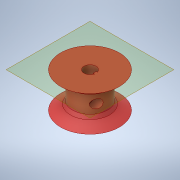
# Autodesk Inventor part: RoundShaftSpoolForArmV01
Saved by Autodesk Inventor 2022.2 (Build 262287010, 287A)
## iProperties
Created: 2019-02-24
Part Number: RoundShaftSpoolForArmV01
Material: PC/ABS Plastic
Document SubType Name: Modeling
Designer: steele
Density: 0.357273 g/cm^3
Appearance: Smooth - Red
holeForString: 0.200 in
stringDiameter: 0.120 in
clearanceForString: 0.080 in
clearanceForHexShaft: 0.020 in
spoolInteriorDiameter: 1.500 in
spoolInteriroRadius: 0.750 in
spoolExteriorDiameter: 2.500 in
spoolExteriorRadius: 1.250 in
hexHoleChamfer: 0.063 in
stringHoleCenterFromHexShaft: 0.360 in
textCircleDiameter: 1.875 in
textHeight: 0.180 in
textDepth: 0.050 in
Author: steele
Autodesk Inventor part; units mm, degrees
(part 1 of 2)
ref_plane "XZ Plane" through (0, 0, 0) normal (0, 1, 0) x (-1, 0, 0)
sketch "Sketch15" plane through (0, 0, 0) normal (0, 0, 1) x (1, 0, 0)
  line L0 (31.75, 0) -> (31.75, 76.2) construction
  line L1 (12.065, 0) -> (31.75, 0)
  line L2 (19.05, 0) -> (19.05, 76.2) construction
  line L3 (0, 76.2) -> (0, 0)
  line L4 (19.05, 19.05) -> (31.75, 19.05) construction
  line L5 (31.75, 0) -> (19.05, 7.3323)
  line L6 (31.75, 38.1) -> (19.05, 30.7677)
  line L7 (19.05, 30.7677) -> (31.75, 30.7677) construction
  line L8 (19.05, 30.7677) -> (19.05, 7.3323)
  line L9 (31.75, 38.1) -> (19.05, 45.4323)
  line L10 (19.05, 45.4323) -> (19.05, 68.8677)
  line L11 (19.05, 68.8677) -> (31.75, 76.2)
  line L12 (31.75, 38.1) -> (19.05, 38.1) construction
  line L13 (19.05, 68.8677) -> (31.75, 68.8677) construction
  line L14 (12.065, 0) -> (0, 0)
  line L15 (31.75, 76.2) -> (0, 76.2)
  dimension "d86" = 76.2
  dimension "d89" = 38.1
  dimension "centerLineForSpool" = 19.05
  dimension "d93" = 30
  dimension "d94" = 30
  dimension "d95" = 30
  dimension "d96" = 30
  dimension "d156" = 31.75
  dimension "d158" = 31.75
  constraints: 32 end point, 9 point on line, 3 horizontal, 2 midpoint, 2 perpendicular, 1 collinear, 1 vertical
  measures "d86" distance of L0.start L0.end
  measures "d89" distance from line of L6.start L1
  measures "centerLineForSpool" distance from line of L4.start L1
  measures "d93" angle of L5 L1
  measures "d94" angle of L6 L7
  measures "d95" angle of L9 L12
  measures "d96" angle of L11 L13
  measures "d156" distance from line of L0.end L3
  measures "d158" distance from line of L0.start L3
revolve "Revolution2" add sketch "Sketch15" angle 360 about axis through (0, 76.2, 0) along (0, -1, 0)
sketch "Sketch16" plane through (0, 0, 0) normal (0, -1, 0) x (1, 0, 0)
  line L0 (-7.6256, 0) -> (-3.8128, 6.604)
  line L1 (-3.8128, 6.604) -> (3.8128, 6.604)
  line L2 (3.8128, 6.604) -> (7.6256, 0)
  line L3 (7.6256, 0) -> (3.8128, -6.604)
  line L4 (3.8128, -6.604) -> (-3.8128, -6.604)
  line L5 (-3.8128, -6.604) -> (-7.6256, 0)
  point P0 (0, 0)
  point P1 (0, 0)
  dimension "d103" = 13.208
  constraints: 12 end point, 1 coincident, 1 horizontal, 13 other
  measures "d103" distance between parallel lines of L1 L4
extrude "Extrusion11" cut sketch "Sketch16" against normal through all
sketch "Sketch17" plane through (0, 0, 0) normal (1, 0, 0) x (0, 1, 0)
  circle A0 centre (57.15, 9.144) radius 2.54
  circle A1 centre (19.05, 9.144) radius 2.54
  line L0 (0, 31.75) -> (0, -31.75) projected
  line L1 (76.2, 31.75) -> (76.2, -31.75) projected
  line L2 (0, 6.604) -> (76.2, 6.604) projected
  point P0 (0, 0)
  point P1 (76.2, -31.75)
  point P2 (69.85, 6.858)
  point P3 (72.39, 6.858)
  dimension "d110" = 19.05
  dimension "d111" = 19.05
  dimension "d112" = 5.08
  constraints: 2 centre point, 1 equal radius, 4 other
  measures "d110" distance from line of A1.centre L0
  measures "d112" diameter of A0
extrude "Extrusion13" cut sketch "Sketch17" along normal through all both and the other way through all
ref_plane "Work Plane4" through (-19.05, 0, 0) normal (1, 0, 0) x (0, 1, 0)
sketch "Sketch22" plane through (-19.05, 0, 0) normal (1, 0, 0) x (0, 1, 0)
  spline S0 degree 8 poles (59.69, 9.144) (59.69, 9.42) (59.6557, 9.6896) (59.59, 9.9488) (59.4956, 10.1945) (59.3753, 10.4241) (59.2322, 10.6353) (59.069, 10.8263) (58.7143, 11.1594) (58.5223, 11.3044) (58.3151, 11.4282) (58.0956, 11.5293) (57.8665, 11.6061) (57.6306, 11.6579) (57.3908, 11.684) (56.8688, 11.684) (56.5895, 11.6484) (56.3166, 11.5781) (56.0542, 11.4743) (55.8066, 11.3384) (55.5778, 11.1726) (55.372, 10.9796) (55.0148, 10.5477) (54.8595, 10.305) (54.7334, 10.0377) (54.6415, 9.75) (54.5882, 9.4472) (54.5771, 9.1354) (54.6105, 8.8213) (54.8033, 8.0702) (55.0037, 7.6667) (55.2756, 7.316) (55.6042, 7.0287) (55.9734, 6.8124) (56.3659, 6.6712) (56.7636, 6.604) (57.4275, 6.604) (57.7064, 6.6386) (57.9825, 6.7085) (58.2515, 6.8141) (58.5088, 6.9552) (58.7493, 7.1318) (58.9675, 7.3429) (59.2831, 7.7498) (59.3961, 7.9265) (59.4931, 8.1154) (59.572, 8.3139) (59.6315, 8.5192) (59.6708, 8.7281) (59.69, 8.9374) (59.69, 9.144) knots 0 0 0 0 0 0 0 0 0 0.12897 0.12897 0.12897 0.12897 0.12897 0.12897 0.12897 0.253758 0.253758 0.253758 0.253758 0.253758 0.253758 0.253758 0.399502 0.399502 0.399502 0.399502 0.399502 0.399502 0.399502 0.544455 0.544455 0.544455 0.544455 0.544455 0.544455 0.544455 0.751871 0.751871 0.751871 0.751871 0.751871 0.751871 0.751871 0.90085 0.90085 0.90085 0.90085 0.90085 0.90085 0.90085 1 1 1 1 1 1 1 1 1 projected
  circle A0 centre (57.15, 9.144) radius 4.7625
  circle A1 centre (57.15, 9.144) radius 2.54 construction
  line L0 (57.15, 6.604) -> (19.05, 6.604) construction
  line L1 (76.2, 31.75) -> (76.2, -31.75) construction
  point P0 (0, 0)
  point P1 (69.85, 6.858)
  point P2 (76.2, -31.75)
  point P3 (72.39, 6.858)
  point P4 (19.05, 6.604)
  dimension "d121" = 19.05
  dimension "d122" = 5.08
  dimension "d125" = 9.525
  constraints: 2 centre point, 1 concentric, 1 vertical alignment, 3 other
  measures "d122" diameter of A1
  measures "d125" diameter of A0
extrude "Extrusion16" cut sketch "Sketch22" along normal blind 11.1125
ref_plane "Work Plane5" through (19.05, 0, 0) normal (1, 0, 0) x (0, 1, 0)
sketch "Sketch23" plane through (19.05, 0, 0) normal (1, 0, 0) x (0, 1, 0)
  line L0 (19.05, 6.604) -> (57.15, 6.604) projected
  circle A0 centre (19.05, 9.144) radius 2.54 construction
  line L1 (0, 31.75) -> (0, -31.75) projected
  circle A1 centre (19.05, 9.144) radius 4.7625
  point P0 (0, 0)
  dimension "d127" = 5.08
  dimension "d128" = 19.05
  dimension "d129" = 9.525
  constraints: 2 centre point, 1 coincident, 1 tangent
  measures "d127" diameter of A0
  measures "d128" distance from line of A0.centre L1
  measures "d129" diameter of A1
extrude "Extrusion17" cut sketch "Sketch23" against normal blind 11.1125
chamfer "Chamfer12" distance 2.3813 angle 45 4 edges at (-19.05, 68.8677, 0) (-19.05, 45.4323, 0) (-19.05, 30.7677, 0) (-19.05, 7.3323, 0)
ref_plane "Work Plane6" through (0, 38.1, 0) normal (0, -1, 0) x (1, 0, 0)
sketch "Sketch26" plane through (0, 0, 0) normal (0, -1, 0) x (1, 0, 0)
  circle A0 centre (0, 0) radius 23.8125 construction
  spline S0 degree 2 poles (-23.6535, 2.0269) (-23.7163, 1.1708) (-24.8247, 0.243) (-25.7608, 0.3118) knots 0 0 0 1 2 2 2
  spline S1 degree 2 poles (-25.7608, 0.3118) (-26.663, 0.378) (-27.6637, 1.4639) (-27.6008, 2.3199) knots 0 0 0 1 2 2 2
  spline S2 degree 2 poles (-27.6008, 2.3199) (-27.5843, 2.5447) (-27.5053, 2.9042) (-27.4499, 3.0673) knots 0 0 0 1 2 2 2
  spline S3 degree 2 poles (-27.4499, 3.0673) (-27.4004, 3.1937) (-27.2456, 3.4888) (-27.1893, 3.5806) knots 0 0 0 1 2 2 2
  line L0 (-27.1893, 3.5806) -> (-26.284, 3.5141)
  line L1 (-26.284, 3.5141) -> (-26.2911, 3.4187)
  spline S4 degree 2 poles (-26.2911, 3.4187) (-26.3578, 3.3524) (-26.5457, 3.1557) (-26.6354, 3.0291) knots 0 0 0 1 2 2 2
  spline S5 degree 2 poles (-26.6354, 3.0291) (-26.7283, 2.9028) (-26.8655, 2.594) (-26.8784, 2.4185) knots 0 0 0 1 2 2 2
  spline S6 degree 2 poles (-26.8784, 2.4185) (-26.8936, 2.2122) (-26.7894, 1.8609) (-26.6377, 1.6919) knots 0 0 0 1 2 2 2
  spline S7 degree 2 poles (-26.6377, 1.6919) (-26.5034, 1.5396) (-26.021, 1.3215) (-25.6853, 1.2969) knots 0 0 0 1 2 2 2
  spline S8 degree 2 poles (-25.6853, 1.2969) (-25.3312, 1.2709) (-24.834, 1.4232) (-24.6749, 1.5663) knots 0 0 0 1 2 2 2
  spline S9 degree 2 poles (-24.6749, 1.5663) (-24.5193, 1.7035) (-24.3664, 2.0576) (-24.353, 2.2392) knots 0 0 0 1 2 2 2
  spline S10 degree 2 poles (-24.353, 2.2392) (-24.3392, 2.4271) (-24.4404, 2.7781) (-24.5087, 2.9008) knots 0 0 0 1 2 2 2
  spline S11 degree 2 poles (-24.5087, 2.9008) (-24.5762, 3.0358) (-24.7252, 3.2418) (-24.7846, 3.3173) knots 0 0 0 1 2 2 2
  line L2 (-24.7846, 3.3173) -> (-24.7783, 3.4035)
  line L3 (-24.7783, 3.4035) -> (-23.8853, 3.338)
  spline S12 degree 2 poles (-23.8853, 3.338) (-23.8438, 3.2296) (-23.7407, 2.9465) (-23.7085, 2.7956) knots 0 0 0 1 2 2 2
  spline S13 degree 2 poles (-23.7085, 2.7956) (-23.6662, 2.6129) (-23.6336, 2.2978) (-23.6535, 2.0269) knots 0 0 0 1 2 2 2
  line L4 (-23.3485, 4.6994) -> (-23.5086, 3.8185)
  line L5 (-23.5086, 3.8185) -> (-26.3367, 4.3326)
  line L6 (-26.3367, 4.3326) -> (-26.1766, 5.2135)
  line L7 (-26.1766, 5.2135) -> (-23.3485, 4.6994)
  line L8 (-26.5756, 5.3143) -> (-26.7452, 4.3817)
  line L9 (-26.7452, 4.3817) -> (-27.4317, 4.5065)
  line L10 (-27.4317, 4.5065) -> (-27.2622, 5.4391)
  line L11 (-27.2622, 5.4391) -> (-26.5756, 5.3143)
  line L12 (-24.6721, 7.7572) -> (-24.6912, 7.6857)
  spline S14 degree 2 poles (-24.6912, 7.6857) (-24.7227, 7.6397) (-24.7907, 7.4565) (-24.8209, 7.3432) knots 0 0 0 1 2 2 2
  spline S15 degree 2 poles (-24.8209, 7.3432) (-24.8567, 7.2089) (-24.8566, 6.8861) (-24.8403, 6.7316) knots 0 0 0 1 2 2 2
  line L13 (-24.8403, 6.7316) -> (-22.9817, 6.2358)
  line L14 (-22.9817, 6.2358) -> (-23.2125, 5.3707)
  line L15 (-23.2125, 5.3707) -> (-25.9899, 6.1116)
  line L16 (-25.9899, 6.1116) -> (-25.7591, 6.9767)
  line L17 (-25.7591, 6.9767) -> (-25.3593, 6.8701)
  spline S16 degree 2 poles (-25.3593, 6.8701) (-25.3971, 6.9441) (-25.5085, 7.1975) (-25.5361, 7.2975) knots 0 0 0 1 2 2 2
  spline S17 degree 2 poles (-25.5361, 7.2975) (-25.5673, 7.4081) (-25.581, 7.6802) (-25.5516, 7.7905) knots 0 0 0 1 2 2 2
  spline S18 degree 2 poles (-25.5516, 7.7905) (-25.5405, 7.8323) (-25.5066, 7.9351) (-25.4925, 7.9761) knots 0 0 0 1 2 2 2
  line L18 (-25.4925, 7.9761) -> (-24.6721, 7.7572)
  spline S19 degree 2 poles (-22.0284, 8.846) (-22.1556, 8.5145) (-22.534, 8.028) (-22.7855, 7.8897) knots 0 0 0 1 2 2 2
  spline S20 degree 2 poles (-22.7855, 7.8897) (-23.0376, 7.7583) (-23.6514, 7.7358) (-24.0088, 7.8729) knots 0 0 0 1 2 2 2
  spline S21 degree 2 poles (-24.0088, 7.8729) (-24.3951, 8.0211) (-24.8413, 8.4701) (-24.9335, 8.7468) knots 0 0 0 1 2 2 2
  spline S22 degree 2 poles (-24.9335, 8.7468) (-25.0244, 9.0099) (-24.9779, 9.6138) (-24.8651, 9.9078) knots 0 0 0 1 2 2 2
  spline S23 degree 2 poles (-24.8651, 9.9078) (-24.78, 10.1298) (-24.5059, 10.5339) (-24.3072, 10.7156) knots 0 0 0 1 2 2 2
  line L19 (-24.3072, 10.7156) -> (-23.5923, 10.4413)
  line L20 (-23.5923, 10.4413) -> (-23.6332, 10.3347)
  spline S24 degree 2 poles (-23.6332, 10.3347) (-23.7021, 10.3016) (-23.8727, 10.2017) (-23.952, 10.1329) knots 0 0 0 1 2 2 2
  spline S25 degree 2 poles (-23.952, 10.1329) (-24.0393, 10.0606) (-24.1959, 9.8594) (-24.2501, 9.7181) knots 0 0 0 1 2 2 2
  spline S26 degree 2 poles (-24.2501, 9.7181) (-24.3728, 9.3982) (-24.0609, 8.8751) (-23.6804, 8.7291) knots 0 0 0 1 2 2 2
  spline S27 degree 2 poles (-23.6804, 8.7291) (-23.2768, 8.5743) (-22.7353, 8.7964) (-22.6158, 9.1077) knots 0 0 0 1 2 2 2
  spline S28 degree 2 poles (-22.6158, 9.1077) (-22.555, 9.2663) (-22.5364, 9.5303) (-22.5551, 9.6367) knots 0 0 0 1 2 2 2
  spline S29 degree 2 poles (-22.5551, 9.6367) (-22.572, 9.7391) (-22.6351, 9.9022) (-22.6618, 9.962) knots 0 0 0 1 2 2 2
  line L21 (-22.6618, 9.962) -> (-22.6209, 10.0687)
  line L22 (-22.6209, 10.0687) -> (-21.9031, 9.7933)
  spline S30 degree 2 poles (-21.9031, 9.7933) (-21.899, 9.7091) (-21.8902, 9.4907) (-21.9018, 9.3828) knots 0 0 0 1 2 2 2
  spline S31 degree 2 poles (-21.9018, 9.3828) (-21.9137, 9.2484) (-21.9609, 9.0218) (-22.0284, 8.846) knots 0 0 0 1 2 2 2
  line L23 (-20.3261, 12.4765) -> (-20.7511, 11.6885)
  line L24 (-20.7511, 11.6885) -> (-21.031, 11.8394)
  spline S32 degree 2 poles (-21.031, 11.8394) (-20.9697, 11.5433) (-20.975, 11.1041) (-21.1025, 10.8677) knots 0 0 0 1 2 2 2
  spline S33 degree 2 poles (-21.1025, 10.8677) (-21.3047, 10.4927) (-22.0074, 10.3279) (-22.4857, 10.5858) knots 0 0 0 1 2 2 2
  line L25 (-22.4857, 10.5858) -> (-24.1326, 11.4739)
  line L26 (-24.1326, 11.4739) -> (-23.7047, 12.2674)
  line L27 (-23.7047, 12.2674) -> (-22.4491, 11.5904)
  spline S34 degree 2 poles (-22.4491, 11.5904) (-22.2535, 11.4849) (-21.9932, 11.3691) (-21.8884, 11.3617) knots 0 0 0 1 2 2 2
  spline S35 degree 2 poles (-21.8884, 11.3617) (-21.7891, 11.3572) (-21.627, 11.4627) (-21.5537, 11.5986) knots 0 0 0 1 2 2 2
  spline S36 degree 2 poles (-21.5537, 11.5986) (-21.5098, 11.6801) (-21.4682, 11.9524) (-21.4875, 12.0856) knots 0 0 0 1 2 2 2
  line L28 (-21.4875, 12.0856) -> (-23.2811, 13.0528)
  line L29 (-23.2811, 13.0528) -> (-22.8561, 13.8409)
  line L30 (-22.8561, 13.8409) -> (-20.3261, 12.4765)
  line L31 (-19.4276, 13.7769) -> (-19.9318, 13.0369)
  line L32 (-19.9318, 13.0369) -> (-23.2209, 15.2776)
  line L33 (-23.2209, 15.2776) -> (-22.7167, 16.0176)
  line L34 (-22.7167, 16.0176) -> (-19.4276, 13.7769)
  spline S37 degree 2 poles (-18.2634, 15.7563) (-18.2637, 15.6357) (-18.2621, 15.4452) (-18.2941, 15.3109) knots 0 0 0 1 2 2 2
  spline S38 degree 2 poles (-18.2941, 15.3109) (-18.3264, 15.1809) (-18.4257, 14.966) (-18.5565, 14.8098) knots 0 0 0 1 2 2 2
  spline S39 degree 2 poles (-18.5565, 14.8098) (-18.8023, 14.5162) (-19.5183, 14.4593) (-19.8166, 14.7091) knots 0 0 0 1 2 2 2
  spline S40 degree 2 poles (-19.8166, 14.7091) (-20.0605, 14.9132) (-20.199, 15.3634) (-20.132, 15.6214) knots 0 0 0 1 2 2 2
  spline S41 degree 2 poles (-20.132, 15.6214) (-20.0654, 15.8837) (-19.7024, 16.4616) (-19.4716, 16.7758) knots 0 0 0 1 2 2 2
  line L35 (-19.4716, 16.7758) -> (-19.4834, 16.7857)
  spline S42 degree 2 poles (-19.4834, 16.7857) (-19.6657, 16.9383) (-20.0313, 16.7854) (-20.2573, 16.5155) knots 0 0 0 1 2 2 2
  spline S43 degree 2 poles (-20.2573, 16.5155) (-20.3584, 16.3947) (-20.5443, 15.9947) (-20.6044, 15.7833) knots 0 0 0 1 2 2 2
  line L36 (-20.6044, 15.7833) -> (-20.654, 15.7241)
  line L37 (-20.654, 15.7241) -> (-21.1867, 16.1701)
  spline S44 degree 2 poles (-21.1867, 16.1701) (-21.1298, 16.2957) (-20.8298, 16.8176) (-20.6356, 17.0496) knots 0 0 0 1 2 2 2
  spline S45 degree 2 poles (-20.6356, 17.0496) (-20.1599, 17.6178) (-19.3451, 17.8215) (-18.9568, 17.4965) knots 0 0 0 1 2 2 2
  line L38 (-18.9568, 17.4965) -> (-17.4583, 16.2419)
  line L39 (-17.4583, 16.2419) -> (-18.029, 15.5601)
  line L40 (-18.029, 15.5601) -> (-18.2634, 15.7563)
  line L41 (-18.6043, 16.0417) -> (-19.0613, 16.4242)
  spline S46 degree 2 poles (-19.0613, 16.4242) (-19.1913, 16.2352) (-19.3457, 15.9979) (-19.395, 15.862) knots 0 0 0 1 2 2 2
  spline S47 degree 2 poles (-19.395, 15.862) (-19.4415, 15.7439) (-19.3969, 15.5375) (-19.2927, 15.4503) knots 0 0 0 1 2 2 2
  spline S48 degree 2 poles (-19.2927, 15.4503) (-19.1388, 15.3215) (-18.8821, 15.3924) (-18.7454, 15.5558) knots 0 0 0 1 2 2 2
  spline S49 degree 2 poles (-18.7454, 15.5558) (-18.6701, 15.6458) (-18.5944, 15.9045) (-18.6043, 16.0417) knots 0 0 0 1 2 2 2
  line L42 (-16.9837, 19.5049) -> (-17.0374, 19.4538)
  spline S50 degree 2 poles (-17.0374, 19.4538) (-17.0882, 19.4311) (-17.2419, 19.3105) (-17.3269, 19.2296) knots 0 0 0 1 2 2 2
  spline S51 degree 2 poles (-17.3269, 19.2296) (-17.4276, 19.1339) (-17.5961, 18.8585) (-17.663, 18.7183) knots 0 0 0 1 2 2 2
  line L43 (-17.663, 18.7183) -> (-16.3373, 17.3245)
  line L44 (-16.3373, 17.3245) -> (-16.9861, 16.7074)
  line L45 (-16.9861, 16.7074) -> (-18.9671, 18.7902)
  line L46 (-18.9671, 18.7902) -> (-18.3183, 19.4073)
  line L47 (-18.3183, 19.4073) -> (-18.0332, 19.1075)
  spline S52 degree 2 poles (-18.0332, 19.1075) (-18.0268, 19.1904) (-17.9893, 19.4646) (-17.9606, 19.5643) knots 0 0 0 1 2 2 2
  spline S53 degree 2 poles (-17.9606, 19.5643) (-17.9295, 19.6749) (-17.799, 19.9141) (-17.7162, 19.9928) knots 0 0 0 1 2 2 2
  spline S54 degree 2 poles (-17.7162, 19.9928) (-17.6849, 20.0226) (-17.6023, 20.0926) (-17.5689, 20.1201) knots 0 0 0 1 2 2 2
  line L48 (-17.5689, 20.1201) -> (-16.9837, 19.5049)
  line L49 (-14.473, 22.9578) -> (-14.5289, 22.9193)
  spline S55 degree 2 poles (-14.5289, 22.9193) (-14.5809, 22.9022) (-14.7894, 22.8184) (-14.8682, 22.7641) knots 0 0 0 1 2 2 2
  spline S56 degree 2 poles (-14.8682, 22.7641) (-15.0919, 22.6099) (-15.1424, 22.335) (-14.9865, 22.1088) knots 0 0 0 1 2 2 2
  line L50 (-14.9865, 22.1088) -> (-14.9742, 22.091)
  line L51 (-14.9742, 22.091) -> (-14.387, 22.4959)
  line L52 (-14.387, 22.4959) -> (-14.033, 21.9824)
  line L53 (-14.033, 21.9824) -> (-14.5948, 21.5951)
  line L54 (-14.5948, 21.5951) -> (-13.3171, 19.742)
  line L55 (-13.3171, 19.742) -> (-14.0543, 19.2338)
  line L56 (-14.0543, 19.2338) -> (-15.3319, 21.0868)
  line L57 (-15.3319, 21.0868) -> (-15.6268, 20.8835)
  line L58 (-15.6268, 20.8835) -> (-15.9808, 21.397)
  line L59 (-15.9808, 21.397) -> (-15.6859, 21.6003)
  line L60 (-15.6859, 21.6003) -> (-15.7315, 21.6664)
  spline S57 degree 2 poles (-15.7315, 21.6664) (-16.0294, 22.0985) (-15.8724, 22.8443) (-15.4097, 23.1633) knots 0 0 0 1 2 2 2
  spline S58 degree 2 poles (-15.4097, 23.1633) (-15.2496, 23.2737) (-14.9568, 23.4419) (-14.8411, 23.4916) knots 0 0 0 1 2 2 2
  line L61 (-14.8411, 23.4916) -> (-14.473, 22.9578)
  spline S59 degree 2 poles (-10.6013, 22.9627) (-10.2664, 22.3365) (-10.5652, 21.2522) (-11.1887, 20.9187) knots 0 0 0 1 2 2 2
  spline S60 degree 2 poles (-11.1887, 20.9187) (-11.8094, 20.5867) (-12.8826, 20.9369) (-13.2176, 21.5631) knots 0 0 0 1 2 2 2
  spline S61 degree 2 poles (-13.2176, 21.5631) (-13.5555, 22.1947) (-13.2497, 23.2792) (-12.629, 23.6112) knots 0 0 0 1 2 2 2
  spline S62 degree 2 poles (-12.629, 23.6112) (-12.0083, 23.9433) (-10.9377, 23.5916) (-10.6013, 22.9627) knots 0 0 0 1 2 2 2
  spline S63 degree 2 poles (-11.407, 22.5247) (-11.5279, 22.7507) (-11.763, 23.0135) (-11.8764, 23.0684) knots 0 0 0 1 2 2 2
  spline S64 degree 2 poles (-11.8764, 23.0684) (-11.9982, 23.1258) (-12.2145, 23.1047) (-12.3261, 23.045) knots 0 0 0 1 2 2 2
  spline S65 degree 2 poles (-12.3261, 23.045) (-12.435, 22.9867) (-12.5715, 22.8296) (-12.5928, 22.6992) knots 0 0 0 1 2 2 2
  spline S66 degree 2 poles (-12.5928, 22.6992) (-12.6143, 22.5757) (-12.5314, 22.2243) (-12.4061, 21.9902) knots 0 0 0 1 2 2 2
  spline S67 degree 2 poles (-12.4061, 21.9902) (-12.2823, 21.7588) (-12.0532, 21.5137) (-11.944, 21.4601) knots 0 0 0 1 2 2 2
  spline S68 degree 2 poles (-11.944, 21.4601) (-11.8347, 21.4065) (-11.6005, 21.4267) (-11.4861, 21.4879) knots 0 0 0 1 2 2 2
  spline S69 degree 2 poles (-11.4861, 21.4879) (-11.3908, 21.5389) (-11.2385, 21.7254) (-11.2223, 21.8391) knots 0 0 0 1 2 2 2
  spline S70 degree 2 poles (-11.2223, 21.8391) (-11.2052, 21.9708) (-11.2788, 22.2851) (-11.407, 22.5247) knots 0 0 0 1 2 2 2
  line L62 (-8.4251, 24.4521) -> (-8.494, 24.4249)
  spline S71 degree 2 poles (-8.494, 24.4249) (-8.5496, 24.4229) (-8.7374, 24.3688) (-8.8465, 24.3257) knots 0 0 0 1 2 2 2
  spline S72 degree 2 poles (-8.8465, 24.3257) (-8.9758, 24.2747) (-9.2353, 24.0827) (-9.3498, 23.9778) knots 0 0 0 1 2 2 2
  line L63 (-9.3498, 23.9778) -> (-8.6439, 22.1885)
  line L64 (-8.6439, 22.1885) -> (-9.4769, 21.8599)
  line L65 (-9.4769, 21.8599) -> (-10.5317, 24.5338)
  line L66 (-10.5317, 24.5338) -> (-9.6988, 24.8624)
  line L67 (-9.6988, 24.8624) -> (-9.547, 24.4775)
  spline S73 degree 2 poles (-9.547, 24.4775) (-9.5099, 24.5519) (-9.3724, 24.792) (-9.3083, 24.8737) knots 0 0 0 1 2 2 2
  spline S74 degree 2 poles (-9.3083, 24.8737) (-9.2379, 24.9645) (-9.0273, 25.1373) (-8.921, 25.1792) knots 0 0 0 1 2 2 2
  spline S75 degree 2 poles (-8.921, 25.1792) (-8.8808, 25.1951) (-8.778, 25.229) (-8.7367, 25.242) knots 0 0 0 1 2 2 2
  line L68 (-8.7367, 25.242) -> (-8.4251, 24.4521)
  line L69 (-6.2391, 23.053) -> (-5.6856, 27.0364)
  line L70 (-5.6856, 27.0364) -> (-4.6604, 27.2312)
  line L71 (-4.6604, 27.2312) -> (-2.6841, 23.7286)
  line L72 (-2.6841, 23.7286) -> (-3.6517, 23.5447)
  line L73 (-3.6517, 23.5447) -> (-4.0306, 24.2647)
  line L74 (-4.0306, 24.2647) -> (-5.2075, 24.041)
  line L75 (-5.2075, 24.041) -> (-5.2988, 23.2317)
  line L76 (-5.2988, 23.2317) -> (-6.2391, 23.053)
  line L77 (-4.366, 24.9049) -> (-4.9834, 26.0699)
  line L78 (-4.9834, 26.0699) -> (-5.1334, 24.7591)
  line L79 (-5.1334, 24.7591) -> (-4.366, 24.9049)
  line L80 (-0.5268, 25.8575) -> (-0.6007, 25.8528)
  spline S76 degree 2 poles (-0.6007, 25.8528) (-0.6543, 25.8679) (-0.8496, 25.8739) (-0.9667, 25.8663) knots 0 0 0 1 2 2 2
  spline S77 degree 2 poles (-0.9667, 25.8663) (-1.1053, 25.8574) (-1.4112, 25.7542) (-1.5524, 25.6894) knots 0 0 0 1 2 2 2
  line L81 (-1.5524, 25.6894) -> (-1.4288, 23.7698)
  line L82 (-1.4288, 23.7698) -> (-2.3223, 23.7123)
  line L83 (-2.3223, 23.7123) -> (-2.5071, 26.5808)
  line L84 (-2.5071, 26.5808) -> (-1.6135, 26.6384)
  line L85 (-1.6135, 26.6384) -> (-1.5869, 26.2255)
  spline S78 degree 2 poles (-1.5869, 26.2255) (-1.5289, 26.2849) (-1.3243, 26.4713) (-1.2383, 26.5295) knots 0 0 0 1 2 2 2
  spline S79 degree 2 poles (-1.2383, 26.5295) (-1.1435, 26.5944) (-0.8901, 26.6942) (-0.7761, 26.7016) knots 0 0 0 1 2 2 2
  spline S80 degree 2 poles (-0.7761, 26.7016) (-0.7329, 26.7044) (-0.6247, 26.7051) (-0.5814, 26.7048) knots 0 0 0 1 2 2 2
  line L86 (-0.5814, 26.7048) -> (-0.5268, 25.8575)
  line L87 (3.3601, 23.6087) -> (3.4861, 25.0389)
  spline S81 degree 2 poles (3.4861, 25.0389) (3.5048, 25.2511) (3.5149, 25.5415) (3.4861, 25.6371) knots 0 0 0 1 2 2 2
  spline S82 degree 2 poles (3.4861, 25.6371) (3.4542, 25.7329) (3.3016, 25.83) (3.1571, 25.8427) knots 0 0 0 1 2 2 2
  spline S83 degree 2 poles (3.1571, 25.8427) (3.0556, 25.8517) (2.8509, 25.7798) (2.7267, 25.7071) knots 0 0 0 1 2 2 2
  line L88 (2.7267, 25.7071) -> (2.5481, 23.6802)
  line L89 (2.5481, 23.6802) -> (1.65, 23.7594)
  line L90 (1.65, 23.7594) -> (1.776, 25.1895)
  spline S84 degree 2 poles (1.776, 25.1895) (1.7945, 25.3987) (1.8017, 25.6925) (1.773, 25.788) knots 0 0 0 1 2 2 2
  spline S85 degree 2 poles (1.773, 25.788) (1.7411, 25.8838) (1.5885, 25.9809) (1.4439, 25.9937) knots 0 0 0 1 2 2 2
  spline S86 degree 2 poles (1.4439, 25.9937) (1.3363, 26.0031) (1.1151, 25.9203) (1.0105, 25.8583) knots 0 0 0 1 2 2 2
  line L91 (1.0105, 25.8583) -> (0.8319, 23.8314)
  line L92 (0.8319, 23.8314) -> (-0.06, 23.91)
  line L93 (-0.06, 23.91) -> (0.1923, 26.7734)
  line L94 (0.1923, 26.7734) -> (1.0842, 26.6948)
  line L95 (1.0842, 26.6948) -> (1.0563, 26.378)
  spline S87 degree 2 poles (1.0563, 26.378) (1.2909, 26.5433) (1.6999, 26.7181) (1.9429, 26.6967) knots 0 0 0 1 2 2 2
  spline S88 degree 2 poles (1.9429, 26.6967) (2.2043, 26.6736) (2.5822, 26.3893) (2.6648, 26.1309) knots 0 0 0 1 2 2 2
  spline S89 degree 2 poles (2.6648, 26.1309) (2.9412, 26.3484) (3.4192, 26.5666) (3.6529, 26.546) knots 0 0 0 1 2 2 2
  spline S90 degree 2 poles (3.6529, 26.546) (3.8529, 26.5284) (4.1585, 26.3744) (4.2548, 26.2357) knots 0 0 0 1 2 2 2
  spline S91 degree 2 poles (4.2548, 26.2357) (4.3626, 26.0868) (4.4492, 25.6979) (4.4223, 25.3934) knots 0 0 0 1 2 2 2
  line L96 (4.4223, 25.3934) -> (4.2581, 23.5296)
  line L97 (4.2581, 23.5296) -> (3.3601, 23.6087)
  line L98 (5.9237, 23.0684) -> (5.0434, 23.2767)
  line L99 (5.0434, 23.2767) -> (5.2751, 24.2561)
  line L100 (5.2751, 24.2561) -> (6.1555, 24.0479)
  line L101 (6.1555, 24.0479) -> (5.9237, 23.0684)
  line L102 (6.3538, 24.8862) -> (5.4734, 25.0944)
  line L103 (5.4734, 25.0944) -> (5.7052, 26.0739)
  line L104 (5.7052, 26.0739) -> (6.5855, 25.8657)
  line L105 (6.5855, 25.8657) -> (6.3538, 24.8862)
  spline S92 degree 2 poles (11.5194, 23.0401) (11.3241, 22.5864) (10.8864, 21.9681) (10.6258, 21.808) knots 0 0 0 1 2 2 2
  spline S93 degree 2 poles (10.6258, 21.808) (10.3693, 21.6495) (9.7559, 21.638) (9.3873, 21.7967) knots 0 0 0 1 2 2 2
  spline S94 degree 2 poles (9.3873, 21.7967) (9.0158, 21.9567) (8.6055, 22.409) (8.544, 22.7112) knots 0 0 0 1 2 2 2
  spline S95 degree 2 poles (8.544, 22.7112) (8.4812, 23.0105) (8.6272, 23.7477) (8.8226, 24.2014) knots 0 0 0 1 2 2 2
  spline S96 degree 2 poles (8.8226, 24.2014) (9.0228, 24.6665) (9.4508, 25.2621) (9.7178, 25.4295) knots 0 0 0 1 2 2 2
  spline S97 degree 2 poles (9.7178, 25.4295) (9.9824, 25.5912) (10.599, 25.5946) (10.9564, 25.4407) knots 0 0 0 1 2 2 2
  spline S98 degree 2 poles (10.9564, 25.4407) (11.3335, 25.2783) (11.7357, 24.8228) (11.796, 24.5178) knots 0 0 0 1 2 2 2
  spline S99 degree 2 poles (11.796, 24.5178) (11.8559, 24.2197) (11.7087, 23.4797) (11.5194, 23.0401) knots 0 0 0 1 2 2 2
  spline S100 degree 2 poles (10.6375, 23.4199) (10.9171, 24.0693) (10.9303, 24.6855) (10.678, 24.7942) knots 0 0 0 1 2 2 2
  spline S101 degree 2 poles (10.678, 24.7942) (10.4256, 24.9028) (9.9841, 24.471) (9.7033, 23.8188) knots 0 0 0 1 2 2 2
  spline S102 degree 2 poles (9.7033, 23.8188) (9.4273, 23.1779) (9.4133, 22.552) (9.6657, 22.4433) knots 0 0 0 1 2 2 2
  spline S103 degree 2 poles (9.6657, 22.4433) (9.9152, 22.3358) (10.3603, 22.7762) (10.6375, 23.4199) knots 0 0 0 1 2 2 2
  line L106 (12.0369, 20.5512) -> (11.2478, 20.9935)
  line L107 (11.2478, 20.9935) -> (11.74, 21.8715)
  line L108 (11.74, 21.8715) -> (12.5291, 21.4292)
  line L109 (12.5291, 21.4292) -> (12.0369, 20.5512)
  spline S104 degree 2 poles (15.6568, 19.6743) (15.4839, 19.4297) (15.0253, 19.1338) (14.7562, 19.1009) knots 0 0 0 1 2 2 2
  spline S105 degree 2 poles (14.7562, 19.1009) (14.4872, 19.068) (13.9226, 19.2213) (13.5948, 19.4529) knots 0 0 0 1 2 2 2
  spline S106 degree 2 poles (13.5948, 19.4529) (13.2486, 19.7013) (12.8296, 20.1676) (12.7174, 20.3566) knots 0 0 0 1 2 2 2
  line L110 (12.7174, 20.3566) -> (13.1967, 21.0348)
  line L111 (13.1967, 21.0348) -> (13.2673, 20.9849)
  spline S107 degree 2 poles (13.2673, 20.9849) (13.3046, 20.9094) (13.3903, 20.7203) (13.4767, 20.5912) knots 0 0 0 1 2 2 2
  spline S108 degree 2 poles (13.4767, 20.5912) (13.5574, 20.4699) (13.7458, 20.2498) (13.8845, 20.1518) knots 0 0 0 1 2 2 2
  spline S109 degree 2 poles (13.8845, 20.1518) (14.0055, 20.0662) (14.3307, 19.9272) (14.4735, 19.9473) knots 0 0 0 1 2 2 2
  spline S110 degree 2 poles (14.4735, 19.9473) (14.581, 19.9657) (14.7603, 20.0697) (14.8512, 20.1982) knots 0 0 0 1 2 2 2
  spline S111 degree 2 poles (14.8512, 20.1982) (14.9296, 20.3092) (14.9493, 20.5297) (14.9101, 20.6292) knots 0 0 0 1 2 2 2
  spline S112 degree 2 poles (14.9101, 20.6292) (14.8541, 20.7747) (14.58, 21.0289) (14.4716, 21.1055) knots 0 0 0 1 2 2 2
  spline S113 degree 2 poles (14.4716, 21.1055) (14.3001, 21.2267) (13.9357, 21.4011) (13.7958, 21.4546) knots 0 0 0 1 2 2 2
  line L112 (13.7958, 21.4546) -> (13.7277, 21.5027)
  line L113 (13.7277, 21.5027) -> (14.9626, 23.25)
  line L114 (14.9626, 23.25) -> (17.0251, 21.7924)
  line L115 (17.0251, 21.7924) -> (16.6099, 21.2049)
  line L116 (16.6099, 21.2049) -> (15.2862, 22.1404)
  line L117 (15.2862, 22.1404) -> (14.9209, 21.6235)
  spline S114 degree 2 poles (14.9209, 21.6235) (14.9875, 21.584) (15.165, 21.4661) (15.2129, 21.4322) knots 0 0 0 1 2 2 2
  spline S115 degree 2 poles (15.2129, 21.4322) (15.4373, 21.2736) (15.7514, 20.9156) (15.8342, 20.7172) knots 0 0 0 1 2 2 2
  spline S116 degree 2 poles (15.8342, 20.7172) (15.9287, 20.4764) (15.8528, 19.9517) (15.6568, 19.6743) knots 0 0 0 1 2 2 2
  line L118 (17.4262, 16.2992) -> (15.3871, 18.2186)
  line L119 (15.3871, 18.2186) -> (15.8124, 18.6705)
  spline S117 degree 2 poles (15.8124, 18.6705) (16.2657, 18.634) (17.0222, 18.6088) (17.3318, 18.6269) knots 0 0 0 1 2 2 2
  spline S118 degree 2 poles (17.3318, 18.6269) (17.7374, 18.6479) (18.2264, 18.8025) (18.3872, 18.9734) knots 0 0 0 1 2 2 2
  spline S119 degree 2 poles (18.3872, 18.9734) (18.5692, 19.1667) (18.5323, 19.5915) (18.3255, 19.7862) knots 0 0 0 1 2 2 2
  spline S120 degree 2 poles (18.3255, 19.7862) (18.2198, 19.8857) (17.9823, 20.0117) (17.8475, 20.0623) knots 0 0 0 1 2 2 2
  spline S121 degree 2 poles (17.8475, 20.0623) (17.7129, 20.1084) (17.4933, 20.1455) (17.4385, 20.1547) knots 0 0 0 1 2 2 2
  line L120 (17.4385, 20.1547) -> (17.3845, 20.2055)
  line L121 (17.3845, 20.2055) -> (17.9538, 20.8103)
  spline S122 degree 2 poles (17.9538, 20.8103) (18.1236, 20.7565) (18.7327, 20.4036) (18.9643, 20.1856) knots 0 0 0 1 2 2 2
  spline S123 degree 2 poles (18.9643, 20.1856) (19.4589, 19.72) (19.5522, 18.8011) (19.1776, 18.4032) knots 0 0 0 1 2 2 2
  spline S124 degree 2 poles (19.1776, 18.4032) (18.947, 18.1581) (18.271, 17.904) (17.7495, 17.886) knots 0 0 0 1 2 2 2
  spline S125 degree 2 poles (17.7495, 17.886) (17.4243, 17.8784) (16.864, 17.9182) (16.7435, 17.9298) knots 0 0 0 1 2 2 2
  line L122 (16.7435, 17.9298) -> (17.9193, 16.8231)
  line L123 (17.9193, 16.8231) -> (17.4262, 16.2992)
  spline S126 degree 2 poles (20.9848, 14.9394) (20.5993, 14.6304) (19.9226, 14.2898) (19.6174, 14.2707) knots 0 0 0 1 2 2 2
  spline S127 degree 2 poles (19.6174, 14.2707) (19.3166, 14.2511) (18.7695, 14.5288) (18.5184, 14.842) knots 0 0 0 1 2 2 2
  spline S128 degree 2 poles (18.5184, 14.842) (18.2655, 15.1576) (18.1154, 15.7496) (18.2029, 16.0453) knots 0 0 0 1 2 2 2
  spline S129 degree 2 poles (18.2029, 16.0453) (18.288, 16.339) (18.7628, 16.9215) (19.1483, 17.2304) knots 0 0 0 1 2 2 2
  spline S130 degree 2 poles (19.1483, 17.2304) (19.5434, 17.5471) (20.2008, 17.8723) (20.5152, 17.8948) knots 0 0 0 1 2 2 2
  spline S131 degree 2 poles (20.5152, 17.8948) (20.8247, 17.9134) (21.3708, 17.627) (21.6141, 17.3235) knots 0 0 0 1 2 2 2
  spline S132 degree 2 poles (21.6141, 17.3235) (21.871, 17.003) (22.0123, 16.412) (21.9224, 16.1144) knots 0 0 0 1 2 2 2
  spline S133 degree 2 poles (21.9224, 16.1144) (21.8355, 15.8231) (21.3582, 15.2387) (20.9848, 14.9394) knots 0 0 0 1 2 2 2
  spline S134 degree 2 poles (20.3842, 15.6886) (20.9359, 16.1308) (21.2367, 16.6688) (21.0649, 16.8832) knots 0 0 0 1 2 2 2
  spline S135 degree 2 poles (21.0649, 16.8832) (20.893, 17.0976) (20.3005, 16.9234) (19.7465, 16.4793) knots 0 0 0 1 2 2 2
  spline S136 degree 2 poles (19.7465, 16.4793) (19.202, 16.0428) (18.8959, 15.4967) (19.0677, 15.2823) knots 0 0 0 1 2 2 2
  spline S137 degree 2 poles (19.0677, 15.2823) (19.2377, 15.0703) (19.8373, 15.2503) (20.3842, 15.6886) knots 0 0 0 1 2 2 2
  line L124 (21.5114, 10.2638) -> (20.5498, 12.0744)
  line L125 (20.5498, 12.0744) -> (21.1361, 12.3858)
  line L126 (21.1361, 12.3858) -> (21.3924, 11.9031)
  line L127 (21.3924, 11.9031) -> (23.5848, 13.0674)
  line L128 (23.5848, 13.0674) -> (23.3284, 13.5501)
  line L129 (23.3284, 13.5501) -> (23.9147, 13.8615)
  line L130 (23.9147, 13.8615) -> (24.8763, 12.0508)
  line L131 (24.8763, 12.0508) -> (24.29, 11.7395)
  line L132 (24.29, 11.7395) -> (24.0337, 12.2221)
  line L133 (24.0337, 12.2221) -> (21.8413, 11.0578)
  line L134 (21.8413, 11.0578) -> (22.0977, 10.5751)
  line L135 (22.0977, 10.5751) -> (21.5114, 10.2638)
  spline S138 degree 2 poles (24.7622, 7.1655) (24.2608, 6.9813) (23.3117, 7.1294) (22.9778, 7.385) knots 0 0 0 1 2 2 2
  spline S139 degree 2 poles (22.9778, 7.385) (22.6959, 7.5973) (22.351, 8.2139) (22.2158, 8.582) knots 0 0 0 1 2 2 2
  line L136 (22.2158, 8.582) -> (21.8049, 9.7007)
  line L137 (21.8049, 9.7007) -> (25.3813, 11.0143)
  line L138 (25.3813, 11.0143) -> (25.788, 9.9071)
  spline S140 degree 2 poles (25.788, 9.9071) (25.9263, 9.5304) (26.0723, 8.8373) (25.9933, 8.4794) knots 0 0 0 1 2 2 2
  spline S141 degree 2 poles (25.9933, 8.4794) (25.896, 8.0457) (25.281, 7.356) (24.7622, 7.1655) knots 0 0 0 1 2 2 2
  spline S142 degree 2 poles (24.4295, 8.0892) (24.7831, 8.2191) (25.198, 8.6478) (25.2484, 8.9492) knots 0 0 0 1 2 2 2
  spline S143 degree 2 poles (25.2484, 8.9492) (25.2799, 9.168) (25.1533, 9.5754) (25.0511, 9.8536) knots 0 0 0 1 2 2 2
  line L139 (25.0511, 9.8536) -> (25.0447, 9.871)
  line L140 (25.0447, 9.871) -> (22.8044, 9.0482)
  line L141 (22.8044, 9.0482) -> (22.8108, 9.0308)
  spline S144 degree 2 poles (22.8108, 9.0308) (22.9215, 8.7294) (23.094, 8.3224) (23.282, 8.1776) knots 0 0 0 1 2 2 2
  spline S145 degree 2 poles (23.282, 8.1776) (23.502, 8.0084) (24.0759, 7.9594) (24.4295, 8.0892) knots 0 0 0 1 2 2 2
  line L142 (25.1133, 5.3864) -> (24.908, 6.2674)
  line L143 (24.908, 6.2674) -> (25.8883, 6.4959)
  line L144 (25.8883, 6.4959) -> (26.0936, 5.6148)
  line L145 (26.0936, 5.6148) -> (25.1133, 5.3864)
  line L146 (23.2941, 4.9624) -> (23.0888, 5.8435)
  line L147 (23.0888, 5.8435) -> (24.0691, 6.0719)
  line L148 (24.0691, 6.0719) -> (24.2744, 5.1909)
  line L149 (24.2744, 5.1909) -> (23.2941, 4.9624)
  line L150 (23.8506, -0.0449) -> (23.7131, 2.4677)
  line L151 (23.7131, 2.4677) -> (24.3759, 2.504)
  line L152 (24.3759, 2.504) -> (24.4198, 1.7024)
  line L153 (24.4198, 1.7024) -> (26.4329, 1.8125)
  line L154 (26.4329, 1.8125) -> (26.3891, 2.6141)
  line L155 (26.3891, 2.6141) -> (27.0087, 2.648)
  spline S146 degree 2 poles (27.0087, 2.648) (27.0183, 2.4723) (27.0837, 2.1264) (27.1387, 2.0243) knots 0 0 0 1 2 2 2
  spline S147 degree 2 poles (27.1387, 2.0243) (27.2069, 1.9075) (27.4209, 1.7831) (27.5757, 1.7792) knots 0 0 0 1 2 2 2
  line L156 (27.5757, 1.7792) -> (27.6213, 0.9468)
  line L157 (27.6213, 0.9468) -> (24.4705, 0.7745)
  line L158 (24.4705, 0.7745) -> (24.5134, -0.0086)
  line L159 (24.5134, -0.0086) -> (23.8506, -0.0449)
  line L160 (23.7608, -1.6322) -> (23.8057, -0.7287)
  line L161 (23.8057, -0.7287) -> (24.811, -0.7787)
  line L162 (24.811, -0.7787) -> (24.7661, -1.6822)
  line L163 (24.7661, -1.6822) -> (23.7608, -1.6322)
  spline S148 degree 2 poles (24.5866, -5.264) (24.2907, -5.2181) (23.8216, -4.9391) (23.6723, -4.7128) knots 0 0 0 1 2 2 2
  spline S149 degree 2 poles (23.6723, -4.7128) (23.5231, -4.4866) (23.4091, -3.9127) (23.4706, -3.5161) knots 0 0 0 1 2 2 2
  spline S150 degree 2 poles (23.4706, -3.5161) (23.539, -3.0955) (23.7701, -2.5127) (23.8893, -2.3282) knots 0 0 0 1 2 2 2
  line L164 (23.8893, -2.3282) -> (24.7101, -2.4555)
  line L165 (24.7101, -2.4555) -> (24.6968, -2.541)
  spline S151 degree 2 poles (24.6968, -2.541) (24.6458, -2.608) (24.5146, -2.7689) (24.4374, -2.9038) knots 0 0 0 1 2 2 2
  spline S152 degree 2 poles (24.4374, -2.9038) (24.3647, -3.0299) (24.2514, -3.2967) (24.2254, -3.4645) knots 0 0 0 1 2 2 2
  spline S153 degree 2 poles (24.2254, -3.4645) (24.2027, -3.611) (24.2229, -3.964) (24.3044, -4.0829) knots 0 0 0 1 2 2 2
  spline S154 degree 2 poles (24.3044, -4.0829) (24.3688, -4.171) (24.5417, -4.2853) (24.6973, -4.3095) knots 0 0 0 1 2 2 2
  spline S155 degree 2 poles (24.6973, -4.3095) (24.8315, -4.3303) (25.0377, -4.2498) (25.1094, -4.1704) knots 0 0 0 1 2 2 2
  spline S156 degree 2 poles (25.1094, -4.1704) (25.2148, -4.0555) (25.3204, -3.6969) (25.3408, -3.5657) knots 0 0 0 1 2 2 2
  spline S157 degree 2 poles (25.3408, -3.5657) (25.373, -3.3583) (25.3669, -2.9543) (25.3526, -2.8052) knots 0 0 0 1 2 2 2
  line L166 (25.3526, -2.8052) -> (25.3653, -2.7228)
  line L167 (25.3653, -2.7228) -> (27.4797, -3.051)
  line L168 (27.4797, -3.051) -> (27.0923, -5.5467)
  line L169 (27.0923, -5.5467) -> (26.3815, -5.4364)
  line L170 (26.3815, -5.4364) -> (26.6301, -3.8346)
  line L171 (26.6301, -3.8346) -> (26.0046, -3.7375)
  spline S158 degree 2 poles (26.0046, -3.7375) (25.9989, -3.8147) (25.9723, -4.0262) (25.9633, -4.0842) knots 0 0 0 1 2 2 2
  spline S159 degree 2 poles (25.9633, -4.0842) (25.9212, -4.3557) (25.7403, -4.7963) (25.5995, -4.9588) knots 0 0 0 1 2 2 2
  spline S160 degree 2 poles (25.5995, -4.9588) (25.426, -5.1506) (24.9222, -5.3161) (24.5866, -5.264) knots 0 0 0 1 2 2 2
  line L172 (26.7614, -7.5002) -> (25.3548, -6.9387)
  line L173 (25.3548, -6.9387) -> (25.4987, -6.4339)
  line L174 (25.4987, -6.4339) -> (26.99, -6.6985)
  line L175 (26.99, -6.6985) -> (26.7614, -7.5002)
  line L176 (26.466, -8.5365) -> (25.0594, -7.9749)
  line L177 (25.0594, -7.9749) -> (25.2033, -7.4702)
  line L178 (25.2033, -7.4702) -> (26.6946, -7.7348)
  line L179 (26.6946, -7.7348) -> (26.466, -8.5365)
  spline S161 degree 2 poles (21.954, -13.5209) (21.1326, -13.0929) (20.65, -11.7273) (21.0467, -10.9661) knots 0 0 0 1 2 2 2
  spline S162 degree 2 poles (21.0467, -10.9661) (21.4448, -10.2022) (22.8486, -9.8266) (23.6591, -10.249) knots 0 0 0 1 2 2 2
  spline S163 degree 2 poles (23.6591, -10.249) (24.4723, -10.6727) (24.9659, -12.0371) (24.5678, -12.801) knots 0 0 0 1 2 2 2
  spline S164 degree 2 poles (24.5678, -12.801) (24.1711, -13.5622) (22.7727, -13.9476) (21.954, -13.5209) knots 0 0 0 1 2 2 2
  spline S165 degree 2 poles (22.4106, -12.6448) (22.7145, -12.8031) (23.2031, -12.9011) (23.3929, -12.8642) knots 0 0 0 1 2 2 2
  spline S166 degree 2 poles (23.3929, -12.8642) (23.5882, -12.8302) (23.8514, -12.6192) (23.9284, -12.4713) knots 0 0 0 1 2 2 2
  spline S167 degree 2 poles (23.9284, -12.4713) (24.0097, -12.3153) (24.0302, -12.0021) (23.9492, -11.8102) knots 0 0 0 1 2 2 2
  spline S168 degree 2 poles (23.9492, -11.8102) (23.872, -11.6376) (23.5037, -11.2821) (23.2025, -11.1251) knots 0 0 0 1 2 2 2
  spline S169 degree 2 poles (23.2025, -11.1251) (22.8903, -10.9625) (22.4154, -10.8717) (22.2201, -10.9057) knots 0 0 0 1 2 2 2
  spline S170 degree 2 poles (22.2201, -10.9057) (22.0249, -10.9397) (21.7603, -11.1535) (21.6832, -11.3013) knots 0 0 0 1 2 2 2
  spline S171 degree 2 poles (21.6832, -11.3013) (21.6047, -11.4519) (21.5879, -11.7982) (21.672, -11.9709) knots 0 0 0 1 2 2 2
  spline S172 degree 2 poles (21.672, -11.9709) (21.7628, -12.1575) (22.093, -12.4792) (22.4106, -12.6448) knots 0 0 0 1 2 2 2
  spline S173 degree 2 poles (19.4081, -16.9657) (18.9823, -16.6433) (18.5942, -15.7646) (18.6288, -15.3455) knots 0 0 0 1 2 2 2
  spline S174 degree 2 poles (18.6288, -15.3455) (18.6551, -14.9936) (18.9877, -14.3702) (19.2244, -14.0576) knots 0 0 0 1 2 2 2
  line L180 (19.2244, -14.0576) -> (19.9438, -13.1074)
  line L181 (19.9438, -13.1074) -> (22.9813, -15.4073)
  line L182 (22.9813, -15.4073) -> (22.2694, -16.3476)
  spline S175 degree 2 poles (22.2694, -16.3476) (22.0271, -16.6676) (21.5228, -17.1649) (21.1789, -17.2918) knots 0 0 0 1 2 2 2
  spline S176 degree 2 poles (21.1789, -17.2918) (20.7614, -17.4442) (19.8488, -17.2993) (19.4081, -16.9657) knots 0 0 0 1 2 2 2
  spline S177 degree 2 poles (20.0057, -16.1866) (20.306, -16.414) (20.8909, -16.5315) (21.1718, -16.4112) knots 0 0 0 1 2 2 2
  spline S178 degree 2 poles (21.1718, -16.4112) (21.3729, -16.3194) (21.6473, -15.9928) (21.8262, -15.7565) knots 0 0 0 1 2 2 2
  line L183 (21.8262, -15.7565) -> (21.8374, -15.7417)
  line L184 (21.8374, -15.7417) -> (19.9346, -14.3011)
  line L185 (19.9346, -14.3011) -> (19.9234, -14.3158)
  spline S179 degree 2 poles (19.9234, -14.3158) (19.7296, -14.5718) (19.4803, -14.9369) (19.4601, -15.1733) knots 0 0 0 1 2 2 2
  spline S180 degree 2 poles (19.4601, -15.1733) (19.4366, -15.4498) (19.7054, -15.9593) (20.0057, -16.1866) knots 0 0 0 1 2 2 2
  line L186 (16.7611, -16.9206) -> (17.3916, -16.2718)
  line L187 (17.3916, -16.2718) -> (18.1134, -16.9733)
  line L188 (18.1134, -16.9733) -> (17.483, -17.622)
  line L189 (17.483, -17.622) -> (16.7611, -16.9206)
  line L190 (18.1008, -18.2224) -> (18.7312, -17.5736)
  line L191 (18.7312, -17.5736) -> (19.4531, -18.275)
  line L192 (19.4531, -18.275) -> (18.8226, -18.9238)
  line L193 (18.8226, -18.9238) -> (18.1008, -18.2224)
  line L194 (12.8482, -20.0942) -> (14.8882, -18.621)
  line L195 (14.8882, -18.621) -> (15.2768, -19.1592)
  line L196 (15.2768, -19.1592) -> (14.626, -19.6291)
  line L197 (14.626, -19.6291) -> (15.8064, -21.2637)
  line L198 (15.8064, -21.2637) -> (16.4572, -20.7937)
  line L199 (16.4572, -20.7937) -> (16.8205, -21.2968)
  spline S181 degree 2 poles (16.8205, -21.2968) (16.6778, -21.3998) (16.4221, -21.6416) (16.3659, -21.7432) knots 0 0 0 1 2 2 2
  spline S182 degree 2 poles (16.3659, -21.7432) (16.3044, -21.8637) (16.3154, -22.111) (16.3958, -22.2433) knots 0 0 0 1 2 2 2
  line L200 (16.3958, -22.2433) -> (15.7199, -22.7314)
  line L201 (15.7199, -22.7314) -> (13.8726, -20.1732)
  line L202 (13.8726, -20.1732) -> (13.2368, -20.6323)
  line L203 (13.2368, -20.6323) -> (12.8482, -20.0942)
  line L204 (11.4639, -20.8762) -> (12.2485, -20.4258)
  line L205 (12.2485, -20.4258) -> (12.7496, -21.2988)
  line L206 (12.7496, -21.2988) -> (11.965, -21.7491)
  line L207 (11.965, -21.7491) -> (11.4639, -20.8762)
  spline S183 degree 2 poles (9.0689, -24.1102) (8.8689, -23.6585) (8.7129, -22.9171) (8.7726, -22.6172) knots 0 0 0 1 2 2 2
  spline S184 degree 2 poles (8.7726, -22.6172) (8.8307, -22.3214) (9.2392, -21.8636) (9.6062, -21.7011) knots 0 0 0 1 2 2 2
  spline S185 degree 2 poles (9.6062, -21.7011) (9.976, -21.5374) (10.5867, -21.5439) (10.8501, -21.7042) knots 0 0 0 1 2 2 2
  spline S186 degree 2 poles (10.8501, -21.7042) (11.1123, -21.8616) (11.5538, -22.4698) (11.7537, -22.9215) knots 0 0 0 1 2 2 2
  spline S187 degree 2 poles (11.7537, -22.9215) (11.9587, -23.3845) (12.1047, -24.1032) (12.046, -24.4129) knots 0 0 0 1 2 2 2
  spline S188 degree 2 poles (12.046, -24.4129) (11.9847, -24.7169) (11.5681, -25.1715) (11.2124, -25.3289) knots 0 0 0 1 2 2 2
  spline S189 degree 2 poles (11.2124, -25.3289) (10.8369, -25.4952) (10.2294, -25.4805) (9.9647, -25.3175) knots 0 0 0 1 2 2 2
  spline S190 degree 2 poles (9.9647, -25.3175) (9.7053, -25.1588) (9.2626, -24.5478) (9.0689, -24.1102) knots 0 0 0 1 2 2 2
  spline S191 degree 2 poles (9.9469, -23.7214) (10.2331, -24.368) (10.6761, -24.7965) (10.9274, -24.6853) knots 0 0 0 1 2 2 2
  spline S192 degree 2 poles (10.9274, -24.6853) (11.1786, -24.574) (11.162, -23.9567) (10.8745, -23.3074) knots 0 0 0 1 2 2 2
  spline S193 degree 2 poles (10.8745, -23.3074) (10.592, -22.6694) (10.1424, -22.2336) (9.8912, -22.3448) knots 0 0 0 1 2 2 2
  spline S194 degree 2 poles (9.8912, -22.3448) (9.6427, -22.4548) (9.6632, -23.0806) (9.9469, -23.7214) knots 0 0 0 1 2 2 2
  line L208 (7.1157, -26.8829) -> (6.8282, -25.3958)
  line L209 (6.8282, -25.3958) -> (7.3307, -25.2442)
  line L210 (7.3307, -25.2442) -> (7.9138, -26.642)
  line L211 (7.9138, -26.642) -> (7.1157, -26.8829)
  line L212 (8.1473, -26.5716) -> (7.8598, -25.0845)
  line L213 (7.8598, -25.0845) -> (8.3623, -24.9329)
  line L214 (8.3623, -24.9329) -> (8.9454, -26.3308)
  line L215 (8.9454, -26.3308) -> (8.1473, -26.5716)
  line L216 (0.5638, -23.86) -> (1.517, -23.773)
  line L217 (1.517, -23.773) -> (1.6705, -25.4549)
  line L218 (1.6705, -25.4549) -> (2.9649, -25.3368)
  line L219 (2.9649, -25.3368) -> (2.8114, -23.6549)
  line L220 (2.8114, -23.6549) -> (3.7646, -23.5679)
  line L221 (3.7646, -23.5679) -> (4.1109, -27.3621)
  line L222 (4.1109, -27.3621) -> (3.1577, -27.4491)
  line L223 (3.1577, -27.4491) -> (3.0309, -26.0593)
  line L224 (3.0309, -26.0593) -> (1.7364, -26.1775)
  line L225 (1.7364, -26.1775) -> (1.8633, -27.5672)
  line L226 (1.8633, -27.5672) -> (0.9101, -27.6542)
  line L227 (0.9101, -27.6542) -> (0.5638, -23.86)
  spline S195 degree 2 poles (-1.2688, -23.7257) (-0.7228, -23.7467) (-0.2403, -24.2164) (-0.2601, -24.7286) knots 0 0 0 1 2 2 2
  line L228 (-0.2601, -24.7286) -> (-0.3118, -26.0707)
  line L229 (-0.3118, -26.0707) -> (0.0306, -26.0839)
  line L230 (0.0306, -26.0839) -> (0.0066, -26.7071)
  line L231 (0.0066, -26.7071) -> (-0.3359, -26.6939)
  line L232 (-0.3359, -26.6939) -> (-0.3675, -27.5145)
  line L233 (-0.3675, -27.5145) -> (-1.2622, -27.48)
  line L234 (-1.2622, -27.48) -> (-1.2306, -26.6594)
  line L235 (-1.2306, -26.6594) -> (-2.0944, -26.626)
  line L236 (-2.0944, -26.626) -> (-2.0704, -26.0028)
  line L237 (-2.0704, -26.0028) -> (-1.2065, -26.0361)
  line L238 (-1.2065, -26.0361) -> (-1.1672, -25.0149)
  spline S196 degree 2 poles (-1.1672, -25.0149) (-1.1613, -24.8638) (-1.1588, -24.6383) (-1.1924, -24.5474) knots 0 0 0 1 2 2 2
  spline S197 degree 2 poles (-1.1924, -24.5474) (-1.226, -24.4565) (-1.4039, -24.3446) (-1.5767, -24.3379) knots 0 0 0 1 2 2 2
  spline S198 degree 2 poles (-1.5767, -24.3379) (-1.6508, -24.3351) (-1.8845, -24.3878) (-1.9318, -24.4107) knots 0 0 0 1 2 2 2
  line L239 (-1.9318, -24.4107) -> (-2.0089, -24.4078)
  line L240 (-2.0089, -24.4078) -> (-1.9846, -23.7784)
  spline S199 degree 2 poles (-1.9846, -23.7784) (-1.8382, -23.7469) (-1.5095, -23.7164) (-1.2688, -23.7257) knots 0 0 0 1 2 2 2
  line L241 (-3.6301, -25.4266) -> (-2.7324, -25.5387)
  line L242 (-2.7324, -25.5387) -> (-2.857, -26.5374)
  line L243 (-2.857, -26.5374) -> (-3.7547, -26.4254)
  line L244 (-3.7547, -26.4254) -> (-3.6301, -25.4266)
  line L245 (-3.3988, -23.5731) -> (-2.5011, -23.6851)
  line L246 (-2.5011, -23.6851) -> (-2.6257, -24.6839)
  line L247 (-2.6257, -24.6839) -> (-3.5234, -24.5719)
  line L248 (-3.5234, -24.5719) -> (-3.3988, -23.5731)
  spline S200 degree 2 poles (-8.6999, -23.4456) (-8.6173, -23.177) (-8.2844, -22.7981) (-8.0453, -22.7037) knots 0 0 0 1 2 2 2
  spline S201 degree 2 poles (-8.0453, -22.7037) (-7.8063, -22.6093) (-7.2331, -22.6047) (-6.8584, -22.72) knots 0 0 0 1 2 2 2
  spline S202 degree 2 poles (-6.8584, -22.72) (-6.4334, -22.8507) (-5.8691, -23.1794) (-5.7045, -23.3269) knots 0 0 0 1 2 2 2
  line L249 (-5.7045, -23.3269) -> (-5.9478, -24.1178)
  line L250 (-5.9478, -24.1178) -> (-6.0363, -24.0905)
  spline S203 degree 2 poles (-6.0363, -24.0905) (-6.1979, -23.9019) (-6.6799, -23.5469) (-6.9042, -23.4779) knots 0 0 0 1 2 2 2
  spline S204 degree 2 poles (-6.9042, -23.4779) (-7.037, -23.4371) (-7.3613, -23.389) (-7.4912, -23.433) knots 0 0 0 1 2 2 2
  spline S205 degree 2 poles (-7.4912, -23.433) (-7.5929, -23.4696) (-7.7486, -23.6187) (-7.7985, -23.781) knots 0 0 0 1 2 2 2
  spline S206 degree 2 poles (-7.7985, -23.781) (-7.8484, -23.9433) (-7.7604, -24.161) (-7.655, -24.2386) knots 0 0 0 1 2 2 2
  spline S207 degree 2 poles (-7.655, -24.2386) (-7.5497, -24.3163) (-7.2248, -24.4259) (-7.098, -24.4649) knots 0 0 0 1 2 2 2
  line L251 (-7.098, -24.4649) -> (-6.9415, -24.513)
  line L252 (-6.9415, -24.513) -> (-7.1385, -25.1534)
  line L253 (-7.1385, -25.1534) -> (-7.2831, -25.1089)
  spline S208 degree 2 poles (-7.2831, -25.1089) (-7.4484, -25.0581) (-7.7378, -25.0014) (-7.8488, -25.0157) knots 0 0 0 1 2 2 2
  spline S209 degree 2 poles (-7.8488, -25.0157) (-7.9607, -25.0329) (-8.1208, -25.1646) (-8.1643, -25.3063) knots 0 0 0 1 2 2 2
  spline S210 degree 2 poles (-8.1643, -25.3063) (-8.1988, -25.4184) (-8.1382, -25.5889) (-8.0762, -25.6499) knots 0 0 0 1 2 2 2
  spline S211 degree 2 poles (-8.0762, -25.6499) (-8.0013, -25.7214) (-7.7743, -25.8236) (-7.6917, -25.849) knots 0 0 0 1 2 2 2
  spline S212 degree 2 poles (-7.6917, -25.849) (-7.5589, -25.8898) (-7.2595, -25.9141) (-7.1142, -25.9039) knots 0 0 0 1 2 2 2
  spline S213 degree 2 poles (-7.1142, -25.9039) (-6.9991, -25.8973) (-6.7367, -25.8423) (-6.6736, -25.8262) knots 0 0 0 1 2 2 2
  line L254 (-6.6736, -25.8262) -> (-6.5969, -25.8498)
  line L255 (-6.5969, -25.8498) -> (-6.8365, -26.6289)
  spline S214 degree 2 poles (-6.8365, -26.6289) (-7.0499, -26.6505) (-7.7336, -26.6049) (-8.0671, -26.5023) knots 0 0 0 1 2 2 2
  spline S215 degree 2 poles (-8.0671, -26.5023) (-8.3917, -26.4024) (-8.8353, -26.1432) (-8.9699, -25.9823) knots 0 0 0 1 2 2 2
  spline S216 degree 2 poles (-8.9699, -25.9823) (-9.1204, -25.81) (-9.1974, -25.3987) (-9.1293, -25.1774) knots 0 0 0 1 2 2 2
  spline S217 degree 2 poles (-9.1293, -25.1774) (-9.0331, -24.8646) (-8.5296, -24.5091) (-8.2136, -24.532) knots 0 0 0 1 2 2 2
  line L256 (-8.2136, -24.532) -> (-8.2028, -24.4966)
  spline S218 degree 2 poles (-8.2028, -24.4966) (-8.3272, -24.4389) (-8.546, -24.2682) (-8.6314, -24.1257) knots 0 0 0 1 2 2 2
  spline S219 degree 2 poles (-8.6314, -24.1257) (-8.7115, -23.9976) (-8.7635, -23.6522) (-8.6999, -23.4456) knots 0 0 0 1 2 2 2
  line L257 (-9.748, -21.7305) -> (-8.9157, -22.0851)
  line L258 (-8.9157, -22.0851) -> (-9.3102, -23.0111)
  line L259 (-9.3102, -23.0111) -> (-10.1425, -22.6565)
  line L260 (-10.1425, -22.6565) -> (-9.748, -21.7305)
  spline S220 degree 2 poles (-13.7721, -21.7687) (-13.5322, -21.3368) (-13.0347, -20.7655) (-12.7594, -20.6324) knots 0 0 0 1 2 2 2
  spline S221 degree 2 poles (-12.7594, -20.6324) (-12.4883, -20.5004) (-11.8768, -20.5505) (-11.526, -20.7454) knots 0 0 0 1 2 2 2
  spline S222 degree 2 poles (-11.526, -20.7454) (-11.1724, -20.9418) (-10.8095, -21.433) (-10.7786, -21.7398) knots 0 0 0 1 2 2 2
  spline S223 degree 2 poles (-10.7786, -21.7398) (-10.7462, -22.0439) (-10.9654, -22.7627) (-11.2053, -23.1945) knots 0 0 0 1 2 2 2
  spline S224 degree 2 poles (-11.2053, -23.1945) (-11.4512, -23.6372) (-11.9367, -24.1869) (-12.2192, -24.3266) knots 0 0 0 1 2 2 2
  spline S225 degree 2 poles (-12.2192, -24.3266) (-12.4987, -24.461) (-13.1125, -24.4026) (-13.4526, -24.2136) knots 0 0 0 1 2 2 2
  spline S226 degree 2 poles (-13.4526, -24.2136) (-13.8116, -24.0142) (-14.1661, -23.5206) (-14.1955, -23.2111) knots 0 0 0 1 2 2 2
  spline S227 degree 2 poles (-14.1955, -23.2111) (-14.2252, -22.9086) (-14.0045, -22.187) (-13.7721, -21.7687) knots 0 0 0 1 2 2 2
  spline S228 degree 2 poles (-12.9327, -22.235) (-13.276, -22.853) (-13.351, -23.4648) (-13.1108, -23.5983) knots 0 0 0 1 2 2 2
  spline S229 degree 2 poles (-13.1108, -23.5983) (-12.8705, -23.7317) (-12.388, -23.3463) (-12.0432, -22.7255) knots 0 0 0 1 2 2 2
  spline S230 degree 2 poles (-12.0432, -22.7255) (-11.7043, -22.1156) (-11.6276, -21.4942) (-11.8678, -21.3608) knots 0 0 0 1 2 2 2
  spline S231 degree 2 poles (-11.8678, -21.3608) (-12.1053, -21.2288) (-12.5923, -21.6223) (-12.9327, -22.235) knots 0 0 0 1 2 2 2
  line L261 (-16.2916, -22.5169) -> (-15.2783, -21.3912)